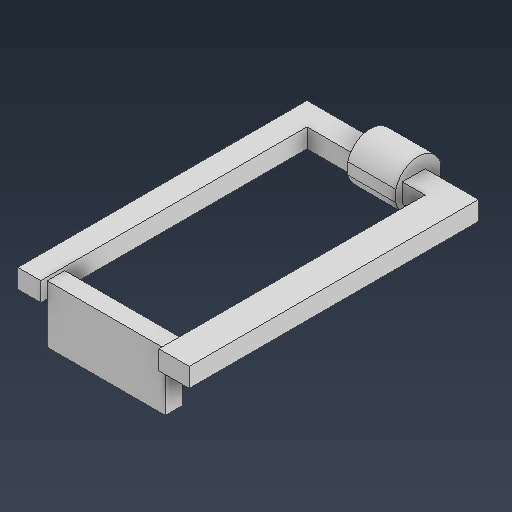
# Autodesk Inventor part: ПАЛЬЧИК ножки врозь
Saved by Autodesk Inventor 2026 (Build 300175000, 175)
## iProperties
Created: 2026-01-11
Part Number: ПАЛЬЧИК ножки врозь
Material: Типовые
Document SubType Name: Modeling
Designer: GameHD
Density: 1 g/cm^3
Appearance: По умолчанию
Author: GameHD
Autodesk Inventor part; units mm, degrees
ref_plane "YZ Plane" through (0, 0, 0) normal (1, 0, 0) x (0, 1, 0)
ref_plane "XZ Plane" through (0, 0, 0) normal (0, 1, 0) x (-1, 0, 0)
ref_plane "XY Plane" through (0, 0, 0) normal (0, 0, 1) x (1, 0, 0)
sketch "Эскиз1" plane through (0, 0, 0) normal (1, 0, 0) x (0, 1, 0)
  line L0 (0, 0) -> (4, 0)
  line L1 (4, 0) -> (4, -125)
  line L2 (4, -125) -> (0, -125)
  line L3 (0, -125) -> (0, 0)
  dimension "d0" = 4
  dimension "d1" = 125
  constraints: 8 end point, 2 parallel, 1 horizontal, 1 perpendicular
  measures "d0" distance of L1.end L2.end
  measures "d1" distance of L0.end L1.end
extrude "Выдавливание1" add sketch "Эскиз1" along normal blind 20
sketch "Эскиз2" plane through (0, 0, 0) normal (0, 0, 1) x (1, 0, 0)
  line L0 (0, 0) -> (0, 4) projected
  line L1 (0, 4) -> (-20.6542, 14.0196)
  line L2 (-20.6542, 14.0196) -> (-22.225, 10.7816)
  line L3 (-22.225, 10.7816) -> (0, 0)
  line L4 (0, 4) -> (20, 4) projected
  line L5 (0, 0) -> (20, 0) projected
  line L6 (10, 4) -> (10, 0)
  line L7 (20, 4) -> (40.6542, 14.0196)
  line L8 (40.6542, 14.0196) -> (42.225, 10.7816)
  line L9 (42.225, 10.7816) -> (20, 0)
  constraints: 14 end point, 2 midpoint, 2 symmetric about line, 1 parallel, 1 perpendicular
extrude "Выдавливание2" add sketch "Эскиз2" against normal blind 20 contours L3 L2 L1 L0 | L6 L4 L7 L8 L9 L5
sketch "Эскиз3" plane through (20, 0, 0) normal (1, 0, 0) x (0, 0, -1)
  circle A0 centre (114.9699, 1.5875) radius 9.6564
  line L0 (125, 0) -> (125, 4) projected
  point P0 (0, 0)
  dimension "d16" = 10.0301
  constraints: 1 centre point
  measures "d16" distance from line of A0.centre L0
extrude "Выдавливание3" add sketch "Эскиз3" against normal blind 20
sketch "Эскиз4" plane through (0, 0, -20) normal (0, 0, -1) x (-1, 0, 0)
  line L0 (-20, 4) -> (-20, 0) projected
  line L1 (-20, 4) -> (-40.6542, 14.0196) projected
  line L2 (-40.6542, 14.0196) -> (-42.225, 10.7816) projected
  line L3 (-42.225, 10.7816) -> (-20, 0) projected
  line L4 (-40.6542, 14.0196) -> (-37.955, 12.7102)
  line L5 (-37.955, 12.7102) -> (-39.5258, 9.4722)
  line L6 (-42.225, 10.7816) -> (-39.5258, 9.4722)
  line L7 (-42.225, 10.7816) -> (-40.6542, 14.0196)
  line L8 (20.6542, 14.0196) -> (0, 4) projected
  line L9 (0, 0) -> (0, 4) projected
  line L10 (0, 0) -> (22.225, 10.7816) projected
  line L11 (22.225, 10.7816) -> (20.6542, 14.0196) projected
  line L12 (20.6542, 14.0196) -> (17.955, 12.7102)
  line L13 (17.955, 12.7102) -> (19.5258, 9.4722)
  line L14 (19.5258, 9.4722) -> (22.225, 10.7816)
  line L15 (20.6542, 14.0196) -> (22.225, 10.7816)
  dimension "d8" = 3
  dimension "d9" = 3
  constraints: 16 end point, 4 point on line, 3 collinear, 1 perpendicular
  measures "d8" distance of L1.end L4.end
  measures "d9" distance of L8.start L12.end
extrude "Выдавливание4" add sketch "Эскиз4" along normal up to surface (105 mm away) contours L5 L3 L2 L1 | L11 L10 L13 L8
sketch "Эскиз5" plane through (39.5258, 9.4722, -125) normal (0, 0, -1) x (-0.8997207, -0.436466, 0)
  line L0 (0, 3.5989) -> (0, 0) projected
  line L1 (0, 0) -> (21.7021, 0) projected
  line L2 (19.9562, 3.5989) -> (21.7021, 0) projected
  line L3 (19.9562, 3.5989) -> (0, 3.5989) projected
  line L4 (53.13, 25.7741) -> (50.3035, 28.0017) projected
  line L5 (50.3035, 28.0017) -> (37.9507, 12.3282) projected
  line L6 (39.6965, 8.7293) -> (37.9507, 12.3282) projected
  line L7 (39.6965, 8.7293) -> (53.13, 25.7741) projected
  line L8 (53.13, 25.7741) -> (50.3035, 28.0017) projected
  line L9 (54.987, 28.1302) -> (53.13, 25.7741) projected
  line L10 (52.1605, 30.3579) -> (54.987, 28.1302) projected
  line L11 (50.3035, 28.0017) -> (52.1605, 30.3579) projected
  line L12 (0, 3.5989) -> (0, 0) projected
  line L13 (-3, 3.5989) -> (0, 3.5989) projected
  line L14 (-3, 0) -> (-3, 3.5989) projected
  line L15 (0, 0) -> (-3, 0) projected
extrude "Выдавливание5" add sketch "Эскиз5" against normal blind 20 contours L3 L2 L1 L0 | L7 L6 L5 L4
sketch "Эскиз6" plane through (0, 4, 0) normal (0, 1, 0) x (1, 0, 0)
  line L0 (0, 105.6197) -> (0, 105) projected
  line L1 (0, 105) -> (0, 20) projected
  line L2 (0, 20) -> (0, 0) projected
  line L3 (0, 0) -> (20, 0) projected
  line L4 (20, 20) -> (20, 0) projected
  line L5 (20, 105) -> (20, 20) projected
  line L6 (20, 105.6197) -> (20, 105) projected
  line L7 (-19.5258, 105) -> (0, 105) projected
  line L8 (0, 105) -> (20, 105)
  line L9 (0, 20) -> (20, 20)
  line L10 (0, 125) -> (20, 125) projected
  line L11 (0, 124.3201) -> (20, 124.3201) projected
  line L12 (20, 125) -> (20, 124.3201) projected
  line L13 (0, 125) -> (0, 124.3201) projected
  line L14 (20, 105.6197) -> (0, 105.6197) projected
  point P0 (0, 0)
  constraints: 4 end point, 1 parallel
extrude "Выдавливание6" cut sketch "Эскиз6" against normal blind 20 contours L14 L6 L8 L0 | L8 L5 L9 L1 | L10 L12 L11 L13
sketch "Эскиз7" plane through (0, 0, -20) normal (0, -1, 0) x (1, 0, 0)
  line L0 (0, 0) -> (0, 20) projected
  line L1 (20, 0) -> (20, 20) projected
  line L2 (0, 20) -> (20, 20)
  line L3 (20, 20) -> (20, 12.7)
  line L4 (20, 12.7) -> (0, 12.7)
  line L5 (0, 12.7) -> (0, 20)
  constraints: 8 end point, 2 parallel, 1 horizontal, 1 perpendicular, 1 point on line
extrude "Выдавливание7" add sketch "Эскиз7" along normal blind 20
sketch "Эскиз8" plane through (0, 0, -105) normal (0, -1, 0) x (1, 0, 0)
  line L0 (20, 97.7) -> (0, 97.7) projected
  line L1 (0, 97.7) -> (0, 85) projected
  line L2 (0, 85) -> (0, 0) projected
  line L3 (0, 0) -> (20, 0) projected
  line L4 (20, 85) -> (20, 0) projected
  line L5 (20, 97.7) -> (20, 85) projected
  line L6 (39.5258, 85) -> (20, 85) projected
  line L7 (0, 85) -> (-19.5258, 85) projected
  line L8 (20, 105) -> (42.225, 105) projected
  line L9 (20, 105) -> (20, 97.7) projected
  line L10 (20, 97.7) -> (20, 85) projected
  line L11 (39.5258, 85) -> (20, 85) projected
  line L12 (39.5258, 85) -> (39.5258, 0) projected
  line L13 (20, 0) -> (39.5258, 0) projected
  line L14 (20, -0.6197) -> (20, 0) projected
  line L15 (20, -19.3201) -> (20, -0.6197) projected
  line L16 (20, -19.3201) -> (20, -20) projected
  line L17 (42.225, -20) -> (20, -20) projected
  line L18 (42.225, 105) -> (42.225, -20) projected
  line L19 (-22.225, 105) -> (0, 105) projected
  line L20 (-22.225, 105) -> (-22.225, -20) projected
  line L21 (-22.225, -20) -> (0, -20) projected
  line L22 (0, -19.3201) -> (0, -20) projected
  line L23 (0, -0.6197) -> (0, -19.3201) projected
  line L24 (0, 0) -> (0, -0.6197) projected
  line L25 (-19.5258, 0) -> (0, 0) projected
  line L26 (-19.5258, 85) -> (-19.5258, 0) projected
  line L27 (0, 85) -> (-19.5258, 85) projected
  line L28 (0, 97.7) -> (0, 85) projected
  line L29 (0, 105) -> (0, 97.7) projected
  line L30 (20, 85) -> (0, 85)
  point P0 (0, 97.7)
  constraints: 3 end point, 1 coincident
extrude "Выдавливание8" cut sketch "Эскиз8" against normal blind 20
sketch "Эскиз9" plane through (20, -20, -7.3) normal (0, 0, -1) x (-1, 0, 0)
  line L0 (-22.225, 25.4) -> (49.2125, 25.4)
  line L1 (49.2125, 25.4) -> (49.2125, 17.4625)
  line L2 (49.2125, 17.4625) -> (-22.225, 17.4625)
  line L3 (-22.225, 17.4625) -> (-22.225, 25.4)
  line L4 (-22.225, 25.4) -> (-9.525, 25.4)
  line L5 (-9.525, 25.4) -> (-9.525, 17.4625)
  line L6 (-9.525, 17.4625) -> (-22.225, 17.4625)
  line L7 (-22.225, 17.4625) -> (-22.225, 25.4)
  line L8 (49.2125, 25.4) -> (39.6875, 25.4)
  line L9 (39.6875, 25.4) -> (39.6875, 17.4625)
  line L10 (39.6875, 17.4625) -> (49.2125, 17.4625)
  line L11 (49.2125, 17.4625) -> (49.2125, 25.4)
  point P0 (20, 20)
  constraints: 24 end point, 6 parallel, 3 horizontal, 3 perpendicular, 2 point on line
extrude "Выдавливание9" add sketch "Эскиз9" along normal blind 110.4875 and the other way blind 10 contours L0 L5 L2 L3 | L0 L1 L2 L9
sketch "Эскиз10" plane through (-19.6875, -2.5375, -117.7875) normal (1, 0, 0) x (0, 0, -1)
  line L0 (-117.7875, -17.4625) -> (-117.7875, 6.5375) projected
  line L1 (-110.4875, -17.4625) -> (-117.7875, -17.4625) projected
  line L2 (-110.4875, -17.4625) -> (-110.4875, 6.5375) projected
  line L3 (-110.4875, 6.5375) -> (-117.7875, 6.5375) projected
  line L4 (-120.4875, 7.9375) -> (0, 7.9375) projected
  line L5 (-120.4875, 0) -> (0, 0) projected
  line L6 (0, 7.9375) -> (-9.525, 7.9375)
  line L7 (-9.525, 7.9375) -> (-9.525, 0)
  line L8 (-9.525, 0) -> (0, 0)
  line L9 (0, 0) -> (0, 7.9375)
  point P0 (-117.7875, 2.5375)
  constraints: 8 end point, 2 parallel, 1 horizontal, 1 perpendicular, 1 point on line
extrude "Выдавливание10" add sketch "Эскиз10" along normal up to surface (49.2125 mm away)
